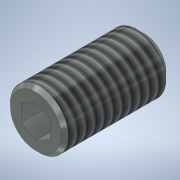
# Autodesk Inventor part: SCREW,SET,CUP POINT,SS, M8X1.25X15MM
Saved by Autodesk Inventor 2022.4 (Build 264492000, 492)
## iProperties
Manager: 605-28684
Category: _
Part Number: SCREW,SET,CUP POINT,SS, M8X1.25X15MM
Material: Stainless Steel, 304L
Document SubType Name: Modeling
Created: 2008-05-22
Designer: Rob.Roddy
Manufacturer: Standard
Standards Organization: Custom
Checked By: 0000225986
Engr Approved By: R
User Status: Released
Description: SCREW,SET,CUP POINT,SS, M8X1.25X15MM
Mfg Approved By: Rob.Roddy
Density: 8.03 g/cm^3
Appearance: Zinc
Mass: 5.604 g
Surface Area: 4.95381 cm^2
Volume: 0.697883 cm^3
Control State: 0
Master: False
Checked Out: False
Shininess: 64.0
Angle Display Precision: 2
Document Length Units: 11269
Document Angle Units: 11279
Document Time Units: 11290
Document Mass Units: 11283
Document Length Units Precision: 3
Document Angle Units Precision: 2
CN_SERVICEABLE: _
FIRST_DESCRIPTION: -
PTC_WM_ITERATION: 2
PTC_WM_ORGANIZATION_ID: CLWC
PTC_WM_LIFECYCLE: CLWC_CAD_LC
CN_MASS: 0.005604
CL_runCount: 1
FinishProperty: ToBeSet
SECOND_DESCRIPTION: _
THIRD_DESCRIPTION: _
Density: 0.0
Volumn: 0.0
Area: 0.0
PropertySet Name: Model Information
Title: SCREW,SET,CUP POINT,SS, M8X1_25X25MM_1FNJ9.ipt
Subject: FSSCPSA080125015
Author: -
Keywords: DEFAULT
Revision Number: A
Autodesk Inventor part; units mm, degrees
ref_plane "YZ Plane" through (0, 0, 0) normal (1, 0, 0) x (0, 1, 0)
ref_plane "XZ Plane" through (0, 0, 0) normal (0, 1, 0) x (-1, 0, 0)
ref_plane "XY Plane" through (0, 0, 0) normal (0, 0, 1) x (1, 0, 0)
sketch "Sketch1" plane through (0, 0, 0) normal (0, 0, 1) x (1, 0, 0)
  line L0 (0, 5.6) -> (0, -5.6) projected
  line L1 (-5.6, 0) -> (5.6, 0) projected
  circle A0 centre (0, 0) radius 4
  dimension "d0" = 8
  constraints: 1 centre point, 1 coincident
  measures "d0" diameter of A0
extrude "Extrusion1" add sketch "Sketch1" along normal blind 15
chamfer "Chamfer1" distance 1 angle 45 1 edges at (-4, 0, 0)
chamfer "Chamfer2" distance 0.5 angle 45 1 edges at (-4, 0, 15)
sketch "Sketch2" plane through (0, 0, 15) normal (0, 0, 1) x (1, 0, 0)
  circle A0 centre (0, 0) radius 3.5 projected
  line L0 (2, -1.1547) -> (0, -2.3094)
  line L1 (0, -2.3094) -> (-2, -1.1547)
  line L2 (-2, -1.1547) -> (-2, 1.1547)
  line L3 (-2, 1.1547) -> (0, 2.3094)
  line L4 (0, 2.3094) -> (2, 1.1547)
  line L5 (2, 1.1547) -> (2, -1.1547)
  line L6 (0, 5.6) -> (0, -5.6) projected
  dimension "d9" = 2
  constraints: 12 end point, 1 coincident, 1 parallel, 11 other
  measures "d9" distance from line of point (0, 0) L5
extrude "Extrusion2" cut sketch "Sketch2" against normal blind 3 contours L6 L1 L2 L3 | L4 L5 L0 L6
thread "Thread1" size "M8x1.25" class "6g" standard "ANSI Metric M Profile" full length
body "Solid1"
